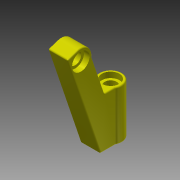
# Autodesk Inventor part: shoulder
Saved by Autodesk Inventor 2013 (Build 170138000, 138)
## iProperties
Created: 2013-07-14
Part Number: shoulder
Material: Generic
Document SubType Name: Modeling
Designer: employee
Density: 1 g/cm^3
Author: employee
Autodesk Inventor part; units mm, degrees
ref_plane "YZ Plane" through (0, 0, 0) normal (1, 0, 0) x (0, 1, 0)
ref_plane "XZ Plane" through (0, 0, 0) normal (0, 1, 0) x (-1, 0, 0)
ref_plane "XY Plane" through (0, 0, 0) normal (0, 0, 1) x (1, 0, 0)
sketch "Sketch1" plane through (0, 0, 0) normal (1, 0, 0) x (0, 1, 0)
  circle A0 centre (-50, 50) radius 7.55
  arc A1 (-38.1519, 53.9839) -> (-61.8481, 46.0161) centre (-50, 50) ccw
  line L0 (0, 0) -> (0, -62.5)
  line L1 (0, -62.5) -> (-25.3601, -62.5)
  line L2 (-25.3601, -62.5) -> (-61.8481, 46.0161)
  line L3 (0, 0) -> (-20, 0)
  line L4 (-20, 0) -> (-38.1519, 53.9839)
  dimension "d0" = 15.1
  dimension "d2" = 50
  dimension "d3" = 50
  dimension "d4" = 25
  dimension "d6" = 62.5
  dimension "d41" = 20
  constraints: 10 end point, 2 centre point, 2 parallel, 2 point on circle, 2 tangent, 1 coincident, 1 perpendicular, 1 vertical
  measures "d0" diameter of A0
  measures "d2" horizontal distance of L0.start A0.centre
  measures "d3" horizontal distance of A0.centre L0.start
  measures "d4" diameter of A1
  measures "d6" distance of L0.start L0.end
  measures "d41" distance of L0.start L3.end
extrude "Extrusion1" add sketch "Sketch1" along normal mid plane 25
sketch "Sketch2" plane through (-12.5, -20, 0) normal (0, 0, 1) x (1, 0, 0)
  circle A0 centre (12.5, 20) radius 12.5
  constraints: 1 centre point, 1 coincident
extrude "Extrusion2" add sketch "Sketch2" against normal up to surface (62.5 mm away)
sketch "Sketch3" plane through (-12.5, -20, 0) normal (0, 0, 1) x (1, 0, 0)
  arc A0 (25, 20) -> (0, 20) centre (12.5, 20) ccw projected
  circle A1 centre (12.5, 20) radius 7.55
  dimension "d11" = 15.1
  constraints: 1 centre point, 1 coincident
  measures "d11" diameter of A1
extrude "Extrusion3" cut sketch "Sketch3" against normal through all
sketch "Sketch4" plane through (-12.5, -20, 0) normal (0, 0, 1) x (1, 0, 0)
  circle A0 centre (12.5, 20) radius 7.55 projected
  arc A1 (25, 20) -> (0, 20) centre (12.5, 20) ccw projected
  circle A2 centre (12.5, 20) radius 11.05
  dimension "d15" = 22.1
  constraints: 1 centre point, 1 coincident
  measures "d15" diameter of A2
extrude "Extrusion4" cut sketch "Sketch4" against normal blind 7
sketch "Sketch5" plane through (12.5, -25.3601, -62.5) normal (0, 0, -1) x (-1, 0, 0)
  circle A0 centre (12.5, 25.3601) radius 7.55 projected
  circle A1 centre (12.5, 25.3601) radius 11.05 projected
extrude "Extrusion5" cut sketch "Sketch5" against normal blind 7
sketch "Sketch7" plane through (12.5, 0, 0) normal (1, 0, 0) x (0, 0, -1)
  circle A0 centre (-50, -50) radius 7.55 projected
  arc A1 (-53.9839, -38.1519) -> (-46.0161, -61.8481) centre (-50, -50) ccw projected
  circle A2 centre (-50, -50) radius 11.05
  dimension "d32" = 22.1
  constraints: 1 centre point, 1 coincident
  measures "d32" diameter of A2
extrude "Extrusion7" cut sketch "Sketch7" against normal blind 7
sketch "Sketch8" plane through (-12.5, 0, 0) normal (-1, 0, 0) x (0, 0, 1)
  circle A0 centre (50, -50) radius 7.55 projected
  circle A1 centre (50, -50) radius 11.05 projected
extrude "Extrusion8" cut sketch "Sketch8" against normal blind 7
sketch "Sketch9" plane through (12.5, -25.3601, -62.5) normal (0, 0, -1) x (-1, 0, 0)
  circle A0 centre (12.5, 25.3601) radius 11.05 projected
  arc A1 (25, 25.3601) -> (0, 25.3601) centre (12.5, 25.3601) ccw projected
  circle A2 centre (12.5, 25.3601) radius 14.05
  dimension "d42" = 3
  constraints: 1 centre point, 1 coincident
  measures "d42" radial gap between concentric circles of A2 A0
extrude "Extrusion9" add sketch "Sketch9" against normal up to surface (62.5 mm away)
sketch "Sketch10" plane through (12.5, 0, 0) normal (1, 0, 0) x (0, 0, -1)
  line L0 (0, -20) -> (-53.9839, -38.1519) projected
  arc A0 (-53.9839, -38.1519) -> (-46.0161, -61.8481) centre (-50, -50) ccw projected
  line L1 (-46.0161, -61.8481) -> (62.5, -25.3601) projected
  circle A1 centre (-50, -50) radius 11.05 projected
  line L2 (-46.0161, -61.8481) -> (-59.3334, -66.326)
  line L3 (-59.3334, -66.326) -> (-63.3173, -54.4779)
  arc A2 (-47.9034, -36.1073) -> (-63.3173, -54.4779) centre (-50, -50) ccw
  point P0 (0, 0)
  dimension "d46" = 3
  constraints: 4 end point, 2 point on circle, 2 tangent, 1 centre point, 1 coincident, 1 collinear, 1 perpendicular, 1 point on line
  measures "d46" radial gap between concentric circles of A2 A1
extrude "Extrusion10" add sketch "Sketch10" against normal up to surface (25 mm away) contours L0 A0 L2 L3 A2
fillet "Fillet3" radius 1.5 20 edges at (-12.5, -60.402, 61.3254) (-12.5, -40.9691, 60.7632) (-12.5, -28.0537, 23.9517) (-12.5, -13.2075, 0) (0, 14.05, 0) (12.5, -13.2075, 0) (12.5, -28.0537, 23.9517) (12.5, -60.402, 61.3254) (12.5, -40.9691, 60.7632) (0, -36.1073, 47.9034) (0, -20, 0) (-12.5, -6.415, -31.25) (12.5, -6.415, -31.25) (0, 14.05, -62.5) (-12.5, -15.8875, -62.5) (12.5, -15.8875, -62.5) (-12.5, -45.8431, -1.5833) (0, -25.3601, -62.5) (12.5, -45.8431, -1.5833) (0, -66.326, 59.3334)
body "Solid1"
